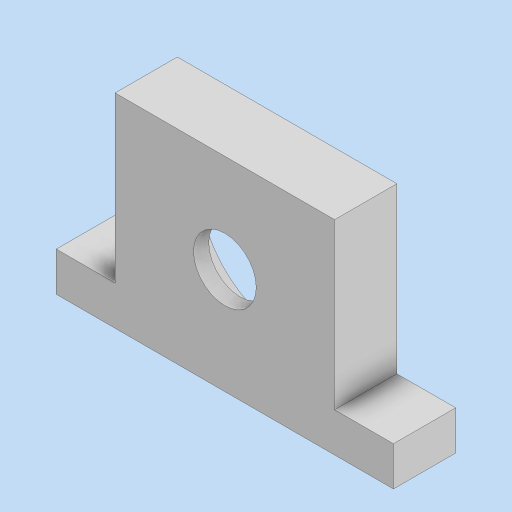
# Autodesk Inventor part: Dudukan PG45
Saved by Autodesk Inventor 2023 (Build 270158000, 158)
## iProperties
Created: 2022-09-10
Part Number: Dudukan PG45
Material: Generic
Document SubType Name: Modeling
Designer: LENOVO
Density: 1 g/cm^3
Appearance: Default
Author: LENOVO
Autodesk Inventor part; units mm, degrees
ref_plane "YZ Plane" through (0, 0, 0) normal (1, 0, 0) x (0, 1, 0)
ref_plane "XZ Plane" through (0, 0, 0) normal (0, 1, 0) x (-1, 0, 0)
ref_plane "XY Plane" through (0, 0, 0) normal (0, 0, 1) x (1, 0, 0)
sketch "Sketch1" plane through (0, 0, 0) normal (0, 0, 1) x (1, 0, 0)
  line L0 (-43, -26) -> (43, -26)
  line L1 (43, -26) -> (43, -16)
  line L2 (28, 26) -> (-28, 26)
  line L3 (-43, -16) -> (-43, -26)
  line L4 (-28, 26) -> (-28, -16)
  line L5 (-28, -16) -> (-43, -16)
  line L6 (28, 26) -> (28, -16)
  line L7 (28, -16) -> (43, -16)
  circle A0 centre (0, 1) radius 22.5
  point P0 (0, 0)
  point P1 (35.5, -16)
  dimension "d4" = 52
  dimension "d5" = 42
  dimension "d6" = 56
  dimension "d7" = 86
  dimension "d8" = 10
  dimension "d9" = 27
  dimension "d10" = 45
  constraints: 16 end point, 2 parallel, 1 centre point, 1 horizontal, 1 midpoint, 1 perpendicular
  measures "d4" distance between parallel lines of L0 L2
  measures "d5" distance of L2.end L4.end
  measures "d6" distance of L2.start L2.end
  measures "d7" distance of L0.start L0.end
  measures "d8" distance from line of L0 point (35.5, -16)
  measures "d9" distance from line of L0 A0.centre
  measures "d10" diameter of A0
extrude "Extrusion1" add sketch "Sketch1" along normal blind 15.875
sketch "Sketch2" plane through (0, 0, 15.875) normal (0, 0, 1) x (1, 0, 0)
  circle A0 centre (0, 1) radius 22.5 projected
  point P0 (0, 0)
extrude "Extrusion2" add sketch "Sketch2" against normal blind 3.875
sketch "Sketch3" plane through (0, 1, 12) normal (0, 0, -1) x (-1, 0, 0)
  circle A0 centre (0, 0) radius 8
  point P0 (0, -1)
  dimension "d15" = 16
  constraints: 1 centre point
  measures "d15" diameter of A0
extrude "Extrusion3" cut sketch "Sketch3" against normal blind 3.875
body "Solid1"
